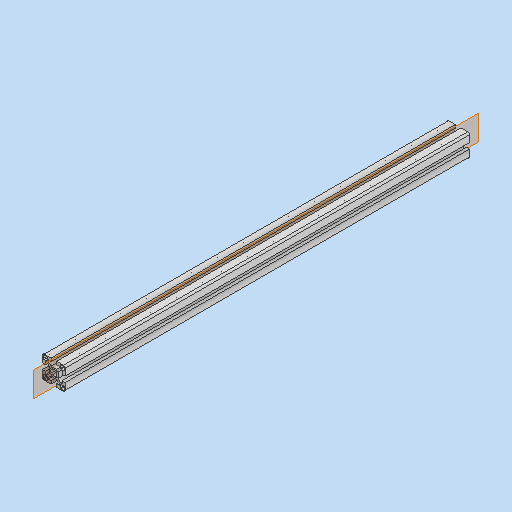
# Autodesk Inventor part: T-SLOT 4040 B-Type 715mm
Saved by Autodesk Inventor 2023.2 (Build 272271000, 271)
## iProperties
Created: 2023-11-21
Part Number: T-SLOT 4040 B-Type 715mm
Material: Generisch
Document SubType Name: Modeling
Designer: Nils Bade
Density: 1 g/cm^3
Appearance: Vorgabe
Author: Nils Bade
Autodesk Inventor part; units mm, degrees
ref_plane "XZ Plane" through (0, 0, 0) normal (0, 1, 0) x (-1, 0, 0)
ref_plane "XY Plane" through (0, 0, 0) normal (0, 0, 1) x (1, 0, 0)
sketch "T-Slot 4040 Base" plane through (0, 0, 0) normal (0, 0, 1) x (1, 0, 0)
  line L0 (-28, 0) -> (28, 0) construction
  line L1 (0, -28) -> (0, 28) construction
  circle A0 centre (0, 0) radius 5.1
  line L2 (-7.5, -7.5) -> (7.5, -7.5)
  line L3 (7.5, -7.5) -> (7.5, 7.5)
  line L4 (7.5, 7.5) -> (-7.5, 7.5)
  line L5 (-7.5, 7.5) -> (-7.5, -7.5)
  line L6 (-7.5, -7.5) -> (7.5, 7.5) construction
  line L7 (7.5, -7.5) -> (-7.5, 7.5) construction
  line L8 (-20, 20) -> (20, 20)
  line L9 (20, 20) -> (20, -20)
  line L10 (20, -20) -> (-20, -20)
  line L11 (-20, -20) -> (-20, 20)
  line L12 (-20, 20) -> (20, -20) construction
  line L13 (20, 20) -> (-20, -20) construction
  line L14 (20, 5) -> (14.5, 5)
  line L15 (14.5, 5) -> (14.5, 10)
  line L16 (14.5, 10) -> (12.4749, 10)
  line L17 (12.4749, 10) -> (7.5, 5.0251)
  line L18 (5, 20) -> (5, 14.5)
  line L19 (5, 14.5) -> (10, 14.5)
  line L20 (10, 14.5) -> (10, 12.4749)
  line L21 (10, 12.4749) -> (5.0251, 7.5)
  line L22 (18.5, 18.5) -> (11.5, 18.5)
  line L23 (11.5, 18.5) -> (11.5, 11.5)
  line L24 (11.5, 11.5) -> (18.5, 11.5)
  line L25 (18.5, 11.5) -> (18.5, 18.5)
  line L26 (18.5, 18.5) -> (11.5, 11.5) construction
  line L27 (11.5, 18.5) -> (18.5, 11.5) construction
  line L28 (3.0732, 1.3088) -> (4.38, 2.6125) construction
  line L29 (5.905, 4.1338) -> (4.1393, 5.9037)
  line L30 (4.1393, 5.9037) -> (2.6122, 4.3802)
  line L31 (1.3075, 3.0787) -> (3.0732, 1.3088) construction
  line L32 (3.0732, 1.3088) -> (4.1393, 5.9037) construction
  line L33 (5.905, 4.1338) -> (1.3075, 3.0787) construction
  line L34 (4.38, 2.6125) -> (5.905, 4.1338)
  line L35 (2.6122, 4.3802) -> (1.3075, 3.0787) construction
  line L36 (-20, 5) -> (-14.5, 5)
  line L37 (-14.5, 5) -> (-14.5, 10)
  line L38 (-14.5, 10) -> (-12.4749, 10)
  line L39 (-12.4749, 10) -> (-7.5, 5.0251)
  line L40 (-5, 20) -> (-5, 14.5)
  line L41 (-5, 14.5) -> (-10, 14.5)
  line L42 (-10, 14.5) -> (-10, 12.4749)
  line L43 (-10, 12.4749) -> (-5.0251, 7.5)
  line L44 (-18.5, 18.5) -> (-11.5, 18.5)
  line L45 (-11.5, 18.5) -> (-11.5, 11.5)
  line L46 (-11.5, 11.5) -> (-18.5, 11.5)
  line L47 (-18.5, 11.5) -> (-18.5, 18.5)
  line L48 (-5.905, 4.1338) -> (-4.1393, 5.9037)
  line L49 (-4.1393, 5.9037) -> (-2.6122, 4.3802)
  line L50 (-4.38, 2.6125) -> (-5.905, 4.1338)
  line L51 (7.5, -7.5) -> (-7.5, -7.5)
  line L52 (20, -5) -> (14.5, -5)
  line L53 (14.5, -5) -> (14.5, -10)
  line L54 (14.5, -10) -> (12.4749, -10)
  line L55 (12.4749, -10) -> (7.5, -5.0251)
  line L56 (5, -20) -> (5, -14.5)
  line L57 (5, -14.5) -> (10, -14.5)
  line L58 (10, -14.5) -> (10, -12.4749)
  line L59 (10, -12.4749) -> (5.0251, -7.5)
  line L60 (18.5, -18.5) -> (11.5, -18.5)
  line L61 (11.5, -18.5) -> (11.5, -11.5)
  line L62 (11.5, -11.5) -> (18.5, -11.5)
  line L63 (18.5, -11.5) -> (18.5, -18.5)
  line L64 (18.5, -18.5) -> (11.5, -11.5) construction
  line L65 (11.5, -18.5) -> (18.5, -11.5) construction
  line L66 (3.0732, -1.3088) -> (4.38, -2.6125) construction
  line L67 (5.905, -4.1338) -> (4.1393, -5.9037)
  line L68 (4.1393, -5.9037) -> (2.6122, -4.3802)
  line L69 (1.3075, -3.0787) -> (3.0732, -1.3088) construction
  line L70 (3.0732, -1.3088) -> (4.1393, -5.9037) construction
  line L71 (5.905, -4.1338) -> (1.3075, -3.0787) construction
  line L72 (4.38, -2.6125) -> (5.905, -4.1338)
  line L73 (2.6122, -4.3802) -> (1.3075, -3.0787) construction
  line L74 (-4.38, -2.6125) -> (-5.905, -4.1338)
  line L75 (-4.1393, -5.9037) -> (-2.6122, -4.3802)
  line L76 (-5.905, -4.1338) -> (-4.1393, -5.9037)
  line L77 (-12.4749, -10) -> (-7.5, -5.0251)
  line L78 (-10, -12.4749) -> (-5.0251, -7.5)
  line L79 (-10, -14.5) -> (-10, -12.4749)
  line L80 (-5, -14.5) -> (-10, -14.5)
  line L81 (-5, -20) -> (-5, -14.5)
  line L82 (-18.5, -18.5) -> (-11.5, -18.5)
  line L83 (-11.5, -18.5) -> (-11.5, -11.5)
  line L84 (-11.5, -11.5) -> (-18.5, -11.5)
  line L85 (-18.5, -11.5) -> (-18.5, -18.5)
  line L86 (-14.5, -10) -> (-12.4749, -10)
  line L87 (-14.5, -5) -> (-14.5, -10)
  line L88 (-20, -5) -> (-14.5, -5)
  point P0 (15, 15)
  point P1 (3.6062, 3.6062)
  point P2 (3.6062, 3.6062)
  point P3 (15, -15)
  point P4 (3.6062, -3.6062)
  point P5 (3.6062, -3.6062)
  dimension "d9" = 10.2
  dimension "d12" = 40
  dimension "d13" = 40
  dimension "d14" = 5.5
  dimension "d15" = 15
  dimension "d16" = 7
  dimension "d17" = 10
  dimension "d20" = 1.75
  dimension "d21" = 7
  dimension "d22" = 2
  dimension "d29" = 1.5
  dimension "d30" = 2.5
  constraints: 174 end point, 64 symmetric about line, 13 midpoint, 12 parallel, 8 perpendicular, 5 point on line, 4 horizontal, 3 point on circle, 1 centre point
  measures "d9" diameter of A0
  measures "d12" distance of L9.end L10.end
  measures "d13" distance of L8.end L9.end
  measures "d14" distance between parallel lines of L9 L15
  measures "d15" distance between parallel lines of L8 L14
  measures "d16" distance between parallel lines of L15 L3
  measures "d17" distance between parallel lines of L0 L16
  measures "d20" distance between parallel lines of L13 L17
  measures "d21" distance of L24.end L23.end
  measures "d22" distance from line of point (3.606, 3.606) L29
  measures "d29" distance between parallel lines of L9 L25
  measures "d30" distance of L29.start L29.end
extrude "Extrusion1" add sketch "T-Slot 4040 Base" along normal blind 715 contours L5 L4 L3 L2 | L2 L78 L79 L80 L81 L10 L11 L88 L87 L86 L77 L5 | L2 L3 L55 L54 L53 L52 L9 L10 L56 L57 L58 L59 | L39 L38 L37 L36 L11 L8 L40 L41 L42 L43 L4 L5 | L3 L4 L21 L20 L19 L18 L8 L9 L14 L15 L16 L17
fillet "Rundung1" radius 1 16 edges at (11.5, 18.5, 357.5) (18.5, 18.5, 357.5) (18.5, 11.5, 357.5) (11.5, 11.5, 357.5) (-11.5, 18.5, 357.5) (-18.5, 18.5, 357.5) (-18.5, 11.5, 357.5) (-11.5, 11.5, 357.5) (-18.5, -11.5, 357.5) (-11.5, -11.5, 357.5) (-11.5, -18.5, 357.5) (-18.5, -18.5, 357.5) (11.5, -18.5, 357.5) (11.5, -11.5, 357.5) (18.5, -11.5, 357.5) (18.5, -18.5, 357.5)
fillet "Rundung2" radius 3 4 edges at (20, 20, 357.5) (20, -20, 357.5) (-20, -20, 357.5) (-20, 20, 357.5)
